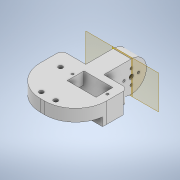
# Autodesk Inventor part: GARRA-base
Saved by Autodesk Inventor 2021 (Build 250183000, 183)
## iProperties
Created: 2023-09-06
Part Number: GARRA-base
Material: Generic
Document SubType Name: Modeling
Designer: PC
Density: 1 g/cm^3
Appearance: Default
Author: PC
Autodesk Inventor part; units mm, degrees
ref_plane "YZ Plane" through (0, 0, 0) normal (1, 0, 0) x (0, 1, 0)
ref_plane "XZ Plane" through (0, 0, 0) normal (0, 1, 0) x (-1, 0, 0)
sketch "Sketch1" plane through (0, 0, 0) normal (1, 0, 0) x (0, 1, 0)
  circle A0 centre (0, 0) radius 12.75
  dimension "d0" = 25.5
  constraints: 1 centre point, 1 coincident
  measures "d0" diameter of A0
extrude "Extrusion1" add sketch "Sketch1" along normal blind 15
ref_plane "Work Plane1" through (0, 0, 0) normal (0, 0, 1) x (1, 0, 0)
ref_plane "Work Plane2" through (0, 0, 0) normal (0, 0, 1) x (1, 0, 0)
sketch "Sketch2" plane through (0, 0, 0) normal (0, 0, 1) x (1, 0, 0)
  line L0 (0, -12.75) -> (0, 12.75) projected
  line L1 (15, -12.75) -> (15, 12.75) projected
  line L2 (0, 12.75) -> (15, 12.75)
  line L3 (15, 12.75) -> (15, 0)
  line L4 (15, 0) -> (0, 0)
  line L5 (0, 0) -> (0, 12.75)
  constraints: 8 end point, 2 parallel, 1 horizontal, 1 midpoint, 1 perpendicular
extrude "Extrusion2" add sketch "Sketch2" along normal blind 12.75
sketch "Sketch3" plane through (0, 0, 12.75) normal (0, 0, 1) x (1, 0, 0)
  line L0 (0, 12.75) -> (0, 0) projected
  line L1 (15, 0) -> (15, 12.75) projected
  line L2 (0, 12.75) -> (15, 12.75)
  line L3 (15, 12.75) -> (15, 2.75)
  line L4 (15, 2.75) -> (0, 2.75)
  line L5 (0, 2.75) -> (0, 12.75)
  dimension "d7" = 10
  constraints: 8 end point, 2 parallel, 1 horizontal, 1 perpendicular, 1 point on line
  measures "d7" distance of L2.end L3.end
extrude "Extrusion3" add sketch "Sketch3" along normal blind 10
sketch "Sketch4" plane through (0, 0, 22.75) normal (0, 0, 1) x (1, 0, 0)
  point P0 (0, 0)
sketch "Sketch5" plane through (0, 12.75, 0) normal (0, 1, 0) x (1, 0, 0)
  line L0 (15, -22.75) -> (0, -22.75) projected
  line L1 (7.5, -22.75) -> (35, -22.75)
  line L2 (7.5, -22.75) -> (-20, -22.75)
  line L3 (35, -22.75) -> (-20, -22.75)
  line L4 (-20, -22.75) -> (-20, -66.25)
  line L5 (-20, -66.25) -> (35, -66.25)
  line L6 (35, -66.25) -> (35, -22.75)
  point P0 (0, 0)
  dimension "d10" = 27.5
  dimension "d11" = 27.5
  dimension "d12" = 55
  dimension "d13" = 43.5
  constraints: 12 end point, 2 parallel, 1 collinear, 1 horizontal, 1 midpoint, 1 perpendicular, 1 point on line
  measures "d10" distance of L1.start L1.end
  measures "d11" distance of L1.start L2.end
  measures "d12" distance of L5.end L4.end
  measures "d13" distance of L4.end L3.end
extrude "Extrusion4" add sketch "Sketch5" against normal blind 10
sketch "Sketch6" plane through (0, 2.75, 12.75) normal (0, -1, 0) x (1, 0, 0)
  line L0 (15, 10) -> (35, 10) projected
  line L1 (35, 10) -> (35, 14)
  line L2 (35, 53.5) -> (35, 10) projected
  line L3 (35, 14) -> (-3, 14)
  line L4 (-3, 14) -> (-3, 31)
  line L5 (-3, 31) -> (35, 31)
  line L6 (35, 31) -> (35, 14)
  line L7 (35, 14) -> (33.5, 14)
  line L8 (33.5, 14) -> (33.5, 15.5)
  line L9 (33.5, 15.5) -> (-1.5, 15.5)
  line L10 (-1.5, 15.5) -> (-1.5, 29.5)
  line L11 (-1.5, 29.5) -> (33.5, 29.5)
  line L12 (33.5, 29.5) -> (33.5, 15.5)
  point P0 (0, -12.75)
  dimension "d16" = 4
  dimension "d17" = 38
  dimension "d18" = 17
  dimension "d19" = 1.5
  dimension "d20" = 1.5
  dimension "d21" = 35
  dimension "d22" = 14
  constraints: 22 end point, 4 parallel, 3 perpendicular, 2 horizontal, 2 point on line
  measures "d16" distance of L0.end L1.end
  measures "d17" distance of L4.end L5.end
  measures "d18" distance of L3.end L4.end
  measures "d19" distance of L1.end L7.end
  measures "d20" distance of L7.end L8.end
  measures "d21" distance of L10.end L11.end
  measures "d22" distance of L9.end L10.end
extrude "Extrusion5" add sketch "Sketch6" along normal blind 7
sketch "Sketch7" plane through (-1.5, 2.75, 42.25) normal (0, -1, 0) x (1, 0, 0)
  line L0 (0, -14) -> (0, 0) projected
  line L1 (0, -7) -> (5.5, -7)
  line L2 (35, 0) -> (35, -14) projected
  line L3 (35, -14) -> (29.5, -14)
  line L4 (35, -14) -> (0, -14) projected
  line L5 (5.5, -7) -> (5.5, 0)
  line L6 (0, 0) -> (35, 0) projected
  line L7 (5.5, 0) -> (29.5, 0)
  line L8 (29.5, 0) -> (29.5, -14)
  line L9 (29.5, -14) -> (5.5, -14)
  line L10 (5.5, -14) -> (5.5, 0)
  point P0 (1.5, -42.25)
  point P1 (5.5, -14)
  point P2 (29.5, 0)
  dimension "d25" = 5.5
  dimension "d26" = 5.5
  constraints: 14 end point, 2 horizontal, 2 parallel, 2 point on line, 1 midpoint, 1 perpendicular, 1 vertical
  measures "d25" distance of L1.start L1.end
  measures "d26" distance of L2.end L3.end
extrude "Extrusion6" cut sketch "Sketch7" against normal blind 20 contours L10 L5 L6 L8 L4
sketch "Sketch8" plane through (33.5, 2.75, 28.25) normal (0, -1, 0) x (1, 0, 0)
  line L0 (-5.5, 14) -> (-5.5, 0) projected
  line L1 (-5.5, 7) -> (-3, 7)
  line L2 (-29.5, 0) -> (-29.5, 14) projected
  line L3 (-29.5, 7) -> (-32, 7)
  circle A0 centre (-3, 7) radius 1
  circle A1 centre (-32, 7) radius 1
  point P0 (-33.5, -28.25)
  dimension "d29" = 2.5
  dimension "d30" = 2.5
  dimension "d31" = 2
  dimension "d32" = 2
  constraints: 4 end point, 2 centre point, 2 coincident, 2 horizontal, 2 midpoint
  measures "d29" distance of L1.start L1.end
  measures "d30" distance of L3.start L3.end
  measures "d31" diameter of A0
  measures "d32" diameter of A1
extrude "Extrusion7" cut sketch "Sketch8" against normal blind 20
sketch "Sketch9" plane through (0, 2.75, 12.75) normal (0, -1, 0) x (1, 0, 0)
  circle A0 centre (1.5, 22.5) radius 1 projected
  line L0 (1.5, 22.5) -> (-8.5, 22.5)
  circle A1 centre (-8.5, 22.5) radius 1.75
  line L1 (-20, 53.5) -> (35, 53.5) projected
  line L2 (-20, 53.5) -> (-20, 48.5)
  line L3 (-20, 10) -> (-20, 53.5) projected
  line L4 (-20, 48.5) -> (1.5, 48.5)
  circle A2 centre (1.5, 48.5) radius 1.75
  line L5 (1.5, 48.5) -> (13.5, 48.5)
  circle A3 centre (13.5, 48.5) radius 1.75
  point P0 (0, -12.75)
  dimension "d35" = 10
  dimension "d36" = 3.5
  dimension "d37" = 5
  dimension "d38" = 21.5
  dimension "d39" = 3.5
  dimension "d40" = 12
  dimension "d41" = 3.5
  constraints: 8 end point, 3 centre point, 3 coincident, 2 horizontal, 1 perpendicular, 1 point on line
  measures "d35" distance of L0.start L0.end
  measures "d36" diameter of A1
  measures "d37" distance of L1.start L2.end
  measures "d38" distance of L2.end L4.end
  measures "d39" diameter of A2
  measures "d40" distance of L5.start L5.end
  measures "d41" diameter of A3
extrude "Extrusion8" cut sketch "Sketch9" against normal blind 12 contours A1 | A2 L5 L4 | L4 L5 A2 | A3
sketch "Sketch10" plane through (15, 0, 0) normal (1, 0, 0) x (0, 0, -1)
  circle A0 centre (0, 0) radius 1.75
  dimension "d44" = 3.5
  constraints: 1 centre point, 1 coincident
  measures "d44" diameter of A0
extrude "Extrusion9" cut sketch "Sketch10" against normal blind 12
sketch "Sketch11" plane through (3, 0, 0) normal (1, 0, 0) x (0, 0, -1)
  circle A0 centre (0, 0) radius 1
  dimension "d47" = 2
  constraints: 1 centre point, 1 coincident
  measures "d47" diameter of A0
extrude "Extrusion10" cut sketch "Sketch11" against normal blind 12
sketch "Sketch12" plane through (0, 0, 0) normal (-1, 0, 0) x (0, 0, 1)
  line L0 (0, 0) -> (6, 0)
  circle A0 centre (0, 0) radius 1.75 projected
  line L1 (0, 0) -> (-6, 0)
  line L2 (-6, 0) -> (0, 0)
  line L3 (0, 0) -> (0, 6)
  line L4 (0, 0) -> (0, -6)
  circle A1 centre (6, 0) radius 1
  circle A2 centre (-6, 0) radius 1
  circle A3 centre (0, 6) radius 1
  circle A4 centre (0, -6) radius 1
  dimension "d50" = 6
  dimension "d51" = 6
  dimension "d52" = 6
  dimension "d53" = 6
  dimension "d54" = 2
  dimension "d55" = 2
  dimension "d56" = 2
  dimension "d57" = 2
  constraints: 10 end point, 4 centre point, 4 coincident, 2 horizontal, 1 collinear, 1 perpendicular, 1 vertical
  measures "d50" distance of L0.start L0.end
  measures "d51" distance of L1.start L1.end
  measures "d52" distance of L1.start L3.end
  measures "d53" distance of L1.start L4.end
  measures "d54" diameter of A1
  measures "d55" diameter of A2
  measures "d56" diameter of A3
  measures "d57" diameter of A4
fillet "Fillet1" radius 25.75 2 edges at (35, 7.75, 66.25) (-20, 7.75, 66.25)
fillet "Fillet2" radius 4 2 edges at (-20, 7.75, 22.75) (35, 7.75, 22.75)
extrude "Extrusion11" cut sketch "Sketch12" against normal blind 20 contours A1 | A2 | A3 | A4
sketch "Sketch13" plane through (0, 12.75, 0) normal (0, 1, 0) x (1, 0, 0)
  point P0 (0, 0)
fillet "Fillet3" radius 11.5 1 edges at (7.5, 2.75, 12.75)
body "Solid1"
